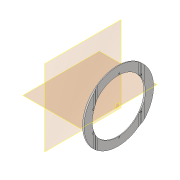
# Autodesk Inventor part: GxFrontplate_base_191210_v02
Saved by Autodesk Inventor 2018 (Build 220112000, 112)
## iProperties
Created: 2019-12-11
Part Number: GxFrontplate_base_191210_v02
Material: Generic
Document SubType Name: Modeling
Designer: pm589
Density: 1 g/cm^3
Appearance: Default
Author: pm589
Autodesk Inventor part; units mm, degrees
ref_plane "XY Plane" through (0, 0, 0) normal (0, 0, 1) x (1, 0, 0)
ref_plane "Work Plane1" through (177.8, 0, 0) normal (1, 0, 0) x (0, 1, 0)
sketch "Sketch1" plane through (177.8, 0, 0) normal (1, 0, 0) x (0, 1, 0)
  circle A0 centre (0, 0) radius 178.9
  circle A1 centre (0, 0) radius 136.9
  dimension "d1" = 357.8
  dimension "d2" = 273.8
  constraints: 2 centre point, 2 coincident
  measures "d1" diameter of A0
  measures "d2" diameter of A1
extrude "Extrusion1" add sketch "Sketch1" along normal blind 3.685
sketch "Sketch2" plane through (181.485, 0, 0) normal (1, 0, 0) x (0, 0, -1)
  line L0 (250.46, 0) -> (-250.46, 0) construction
  line L1 (0, -250.46) -> (0, 250.46) construction
  circle A0 centre (0, 0) radius 141.9 construction
  line L2 (0, 0) -> (-131.5488, 53.2026) construction
  line L3 (0, 0) -> (5.6947, 141.7857) construction
  line L4 (0, 0) -> (115.2635, 82.7643) construction
  point P0 (-131.5488, -53.2026)
  point P1 (5.6947, -141.7857)
  point P2 (115.2635, -82.7643)
  dimension "d5" = 283.8
  dimension "d6" = 22.02
  dimension "d7" = 92.3
  dimension "d8" = 144.32
  constraints: 6 end point, 3 point on circle, 3 symmetric about line, 1 centre point, 1 coincident
  measures "d5" diameter of A0
  measures "d6" angle of L2 L0
  measures "d7" angle of L3 L0
  measures "d8" angle of L0 L4
hole "Hole1" at (181.485, 53.2026, 131.5488) at (181.485, 141.7857, -5.6947) at (181.485, 82.7643, -115.2635) at (181.485, -53.2026, 131.5488) at (181.485, -141.7857, -5.6947) at (181.485, -82.7643, -115.2635) direction (-1, 0, 0) diameter 4 end through all countersink diameter 8 countersink angle 90
sketch "Sketch3" plane through (181.485, 0, 0) normal (1, 0, 0) x (0, 0, -1)
  circle A0 centre (5.6947, -141.7857) radius 4 projected
  circle A1 centre (115.2635, 82.7643) radius 4 projected
  circle A2 centre (-131.5488, 53.2026) radius 4 projected
  circle A3 centre (5.6947, 141.7857) radius 4 projected
  circle A4 centre (-131.5488, -53.2026) radius 4 projected
  circle A5 centre (115.2635, -82.7643) radius 4 projected
  circle A6 centre (0, 0) radius 136.9 projected
  circle A7 centre (0, 0) radius 178.9 projected
extrude "Extrusion2" add sketch "Sketch3" along normal blind 4
sketch "Sketch4" plane through (0, 0, 0) normal (0, 1, 0) x (-1, 0, 0)
  line L0 (-185.485, 178.9) -> (-185.485, -178.9) construction
  line L1 (-177.8, -178.9) -> (-177.8, 178.9) construction
  line L2 (44.297, 0) -> (-265.782, 0) construction
  line L3 (-181.485, 0) -> (-181.485, 104.7583) construction
  line L4 (-185.485, 0) -> (-185.485, 125) construction
  line L5 (-182.8356, 115.0648) -> (-184.1344, 119.9352) construction
  arc A0 (-181.485, 104.7583) -> (-182.8356, 115.0648) centre (-221.485, 104.7583) ccw
  line L6 (-185.485, 130.2417) -> (-185.485, 178.9) construction
  arc A1 (-185.485, 130.2417) -> (-184.1344, 119.9352) centre (-145.485, 130.2417) ccw
  line L7 (-182.8356, 115.0648) -> (-184.1344, 119.9352)
  line L8 (-182.8356, -115.0648) -> (-184.1344, -119.9352) construction
  arc A2 (-182.8356, -115.0648) -> (-181.485, -104.7583) centre (-221.485, -104.7583) ccw
  arc A3 (-184.1344, -119.9352) -> (-185.485, -130.2417) centre (-145.485, -130.2417) ccw
  line L9 (-182.8356, -115.0648) -> (-184.1344, -119.9352)
  line L10 (-181.485, 104.7583) -> (-181.485, -104.7583)
  line L11 (-185.485, -130.2417) -> (-185.485, 130.2417)
  line L12 (-185.485, 127.5488) -> (-185.485, 135.5488) projected
  point P0 (0, 0)
  point P1 (-181.485, 110)
  dimension "d18" = 4
  dimension "d19" = 125
  dimension "d20" = 110
  dimension "d21" = 40
  dimension "d22" = 40
  constraints: 18 end point, 8 point on circle, 7 point on line, 6 symmetric about line, 5 tangent, 4 centre point, 3 collinear, 1 midpoint, 1 parallel, 1 vertical, 2 other
  measures "d18" distance between parallel lines of L0 L3
  measures "d19" distance from line of L2 L4.end
  measures "d20" distance from line of L2 point (-181.485, 110)
  measures "d21" radius of A0
  measures "d22" radius of A1
extrude "Extrusion3" cut sketch "Sketch4" along normal through all both and the other way through all
equation "\"d1\" = gxfront_OD"
equation "\"d2\" = gxfront_ID"
equation "\"d3\" = gxfront_t_total"
equation "\"d5\" = gxfront_d_holpos"
equation "\"d6\" = gxfront_a_hol_1"
equation "\"d7\" = gxfront_a_hol_2"
equation "\"d8\" = gxfront_a_hol_3"
equation "\"d9\" = gxfront_d_hol"
equation "\"d11\" = gxfront_d_holcs"
equation "\"d16\" = gxfront_t_extra"
equation "\"d18\" = gxfront_t_extra"
equation "\"d19\" = gxfront_z_extra"
equation "\"d20\" = gxfront_z_flat"
equation "\"d21\" = gxfront_rfillet_zfair"
equation "\"d22\" = gxfront_rfillet_zfair"
equation "\"d23\" = gxfront_t_extra"
equation "\"gxfront_ID\" = 273.8"
equation "\"gxfront_OD\" = 357.8"
equation "\"gxfront_xbot\" = 177.8"
equation "\"gxfront_tbase\" = 1"
equation "\"gxfront_w_wire\" = 1.074"
equation "\"gxfront_t_total\" = 3.685"
equation "\"gxfront_d_holpos\" = 283.8"
equation "\"gxfront_d_hol\" = 4"
equation "\"gxfront_a_hol_1\" = 22.02deg"
equation "\"gxfront_a_hol_2\" = 92.3deg"
equation "\"gxfront_a_hol_3\" = 144.32deg"
equation "\"d0\" = gxfront_xbot"
equation "\"gxfront_d_holcs\" = 8"
equation "\"gxfront_z_extra\" = 125"
equation "\"gxfront_z_flat\" = 110"
equation "\"gxfront_t_extra\" = 4"
equation "\"gxfront_rfillet_zfair\" = 40"
equation "\"gxfront_t_total_offset\" = 0.5"
body "Solid1"
